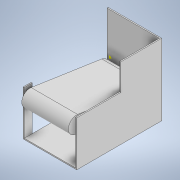
# Autodesk Inventor part: ShootingMech_Housing5
Saved by Autodesk Inventor 2020 (Build 240168000, 168)
## iProperties
Created: 2022-01-22
Part Number: ShootingMech_Housing5
Material: Generic
Document SubType Name: Modeling
Designer: danie
Density: 1 g/cm^3
Appearance: Default
Author: danie
Autodesk Inventor part; units mm, degrees
ref_plane "YZ Plane" through (0, 0, 0) normal (1, 0, 0) x (0, 1, 0)
ref_plane "XZ Plane" through (0, 0, 0) normal (0, 1, 0) x (-1, 0, 0)
ref_plane "XY Plane" through (0, 0, 0) normal (0, 0, 1) x (1, 0, 0)
sketch "Sketch3" plane through (0, 0, 0) normal (1, 0, 0) x (0, 1, 0)
  line L0 (0, 0) -> (232.918, 0) construction
  line L1 (0, 0) -> (208.28, 0) construction
  line L2 (0, 0) -> (194.818, 0) construction
  line L3 (0, 0) -> (156.718, 0) construction
  line L4 (14.398, 96.339) -> (-14.398, -96.339) construction
  line L5 (-7.5829, 99.6241) -> (-36.3788, -93.054)
  line L6 (7.5829, -99.6241) -> (36.3788, 93.054)
  arc A0 (36.3788, 93.054) -> (-7.5829, 99.6241) centre (14.398, 96.339) ccw
  arc A1 (-36.3788, -93.054) -> (7.5829, -99.6241) centre (-14.398, -96.339) ccw
  line L7 (0, 0) -> (194.818, 0) construction
  line L8 (33.2387, 93.5233) -> (4.4428, -99.1548)
  arc A2 (-33.2387, -93.5233) -> (4.4428, -99.1548) centre (-14.398, -96.339) ccw
  line L9 (-33.2387, -93.5233) -> (-4.4428, 99.1548)
  arc A3 (33.2387, 93.5233) -> (-4.4428, 99.1548) centre (14.398, 96.339) ccw
  ellipse E0 centre (-14.398, -96.339) end of major axis (-17.2137, -115.1798) minor radius 19.05
  ellipse E1 centre (14.398, 96.339) end of major axis (33.2387, 93.5233) minor radius 19.05
  dimension "d23" = 97.409
  dimension "d24" = 98.5
  dimension "d25" = 44.45
  dimension "d26" = 3.175
  constraints: 22 end point, 8 point on circle, 5 horizontal, 4 centre point, 4 tangent, 2 coincident, 2 parallel, 1 equal length, 1 midpoint, 10 other
  measures "d23" distance of L0.start L4.end
  measures "d24" angle of L4 L7
  measures "d25" diameter of A1
  measures "d26" distance between parallel lines of L6 L8
extrude "Extrusion3" add sketch "Sketch3" along normal blind 127 contours A0 L6 A1 L5 | E1 A3 | A2 E0
sketch "Sketch4" plane through (127, 0, 0) normal (1, 0, 0) x (0, 0, -1)
  arc A0 (-99.1548, -4.4428) -> (-93.5233, 33.2387) centre (-96.339, 14.398) ccw projected
  circle A1 centre (-96.339, 14.398) radius 3.175
  line L0 (-96.339, 14.398) -> (96.339, -14.398) construction
  line L1 (-96.339, 14.398) -> (98.479, 14.398) construction
  circle A2 centre (96.339, -14.398) radius 3.175
  point P0 (0, 0)
  dimension "d27" = 6.35
  dimension "d28" = 194.818
  dimension "d29" = 8.5
  dimension "d30" = 6.35
  constraints: 4 end point, 2 centre point, 2 coincident, 1 equal length, 1 horizontal
  measures "d27" diameter of A1
  measures "d28" distance of L0.start L0.end
  measures "d29" angle of L0 L1
  measures "d30" diameter of A2
extrude "Extrusion4" add sketch "Sketch4" along normal blind 6.35
sketch "Sketch5" plane through (133.35, 14.398, 96.339) normal (1, 0, 0) x (0, 0, -1)
  line L0 (219.7276, -97.9907) -> (219.7276, 96.8375)
  line L1 (219.7276, 96.8375) -> (-8.8724, 96.8375)
  line L2 (-8.8724, 96.8375) -> (-8.8724, -97.9907)
  line L3 (-8.8724, -97.9907) -> (219.7276, -97.9907)
  line L4 (219.7276, -97.9907) -> (414.5558, -97.9907) construction
  line L5 (-8.8724, 96.8375) -> (111.7776, 96.8375)
  line L6 (111.7776, 96.8375) -> (111.7776, 24.8285)
  line L7 (111.7776, 24.8285) -> (-8.8724, 24.8285)
  line L8 (-8.8724, 24.8285) -> (-8.8724, 96.8375)
  point P0 (96.339, -14.398)
  dimension "d33" = 90
  dimension "d34" = 228.6
  dimension "d50" = 120.65
  dimension "d51" = 72.009
  constraints: 18 end point, 4 parallel, 3 perpendicular, 1 horizontal, 1 point on line
  measures "d33" angle of L4 L0
  measures "d34" distance of L1.end L0.end
  measures "d50" distance of L1.end L5.end
  measures "d51" distance of L5.end L6.end
extrude "Extrusion5" add sketch "Sketch5" along normal blind 3.175 contours L3 L2 L7 L6 L1 L0
sketch "Sketch6" plane through (133.35, 14.398, 96.339) normal (-1, 0, 0) x (0, 0, 1)
  line L0 (8.8724, -97.9907) -> (-219.7276, -97.9907) projected
  line L1 (-219.7276, -97.9907) -> (8.8724, -97.9907)
  line L2 (8.8724, -97.9907) -> (8.8724, -94.8157)
  line L3 (8.8724, -94.8157) -> (-219.7276, -94.8157)
  line L4 (-219.7276, -94.8157) -> (-219.7276, -97.9907)
  point P0 (-96.339, -14.398)
  dimension "d37" = 3.175
  constraints: 8 end point, 3 equal length, 1 perpendicular
  measures "d37" distance of L2.end L0.start
extrude "Extrusion6" add sketch "Sketch6" along normal blind 139.7
sketch "Sketch7" plane through (0, 0, 0) normal (-1, 0, 0) x (0, 0, 1)
  circle A0 centre (96.339, 14.398) radius 3.175 projected
  circle A1 centre (96.339, 14.398) radius 3.175
  point P0 (0, 0)
  dimension "d40" = 6.35
  constraints: 1 centre point, 1 coincident
  measures "d40" diameter of A1
extrude "Extrusion7" add sketch "Sketch7" along normal blind 6.35
sketch "Sketch8" plane through (-6.35, 14.398, 96.339) normal (-1, 0, 0) x (0, 0, 1)
  arc A0 (3.2851, -21.9809) -> (-3.2851, 21.9809) centre (0, 0) ccw construction
  line L0 (0, 0) -> (0, 25.4) construction
  line L1 (0, 25.4) -> (12.7, 25.4) construction
  line L2 (12.7, 25.4) -> (-12.7, 25.4) construction
  line L3 (-12.7, 25.4) -> (-12.7, -97.9907) construction
  line L4 (-12.7, -97.9907) -> (12.7, -97.9907) construction
  line L5 (12.7, -97.9907) -> (12.7, 25.4) construction
  line L6 (8.8724, 24.8285) -> (8.8724, -94.8157) projected
  line L7 (8.8724, 25.4) -> (8.8724, -97.9907)
  line L8 (8.8724, -97.9907) -> (-12.7, -97.9907)
  line L9 (-12.7, -97.9907) -> (-12.7, 25.4)
  line L10 (-111.7776, 24.8285) -> (8.8724, 24.8285) projected
  line L11 (-12.7, 24.8285) -> (8.8724, 24.8285)
  line L12 (-12.7, 24.8285) -> (8.8724, 24.8285) construction
  point P0 (-96.339, -14.398)
  point P1 (8.8724, 96.8375)
  point P2 (8.8724, -94.8157)
  dimension "d43" = 25.4
  dimension "d44" = 12.7
  dimension "d45" = 25.4
  dimension "d52" = 0
  constraints: 22 end point, 4 point on line, 3 horizontal, 3 parallel, 2 collinear, 1 perpendicular, 1 vertical
  measures "d43" distance of L0.start L0.end
  measures "d44" distance of L0.end L1.end
  measures "d45" distance of L1.end L2.end
  measures "d52" distance between parallel lines of L11 L12
extrude "Extrusion8" add sketch "Sketch8" along normal blind 3.175
sketch "Sketch9" plane through (136.525, -83.5928, -123.3885) normal (0, 0, -1) x (-1, 0, 0)
  point P0 (136.525, 83.5928)
sketch "Sketch10" plane through (136.525, -83.5928, -123.3885) normal (0, 0, -1) x (-1, 0, 0)
  line L0 (142.875, 0) -> (146.05, 0) projected
  line L1 (142.875, 0) -> (0, 0) projected
  line L2 (146.05, 0) -> (0, 0)
  line L3 (0, 0) -> (0, 194.8282)
  line L4 (0, 194.8282) -> (146.05, 194.8282)
  line L5 (146.05, 194.8282) -> (146.05, 0)
  point P0 (136.525, 83.5928)
  constraints: 8 end point, 2 parallel, 1 collinear, 1 perpendicular
extrude "Extrusion9" add sketch "Sketch10" along normal blind 3.175
body "Solid2"
